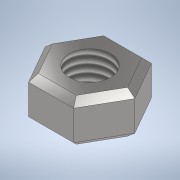
# Autodesk Inventor part: 6-luomu
Saved by Autodesk Inventor 2022 (Build 260153000, 153)
## iProperties
Created: 2023-01-24
Part Number: 6-luomu
Material: 不锈钢
Document SubType Name: Modeling
Designer: Lzy18
Density: 8 g/cm^3
Appearance: 半抛光
Author: Lzy18
Autodesk Inventor part; units mm, degrees
ref_plane "YZ Plane" through (0, 0, 0) normal (1, 0, 0) x (0, 1, 0)
ref_plane "XZ Plane" through (0, 0, 0) normal (0, 1, 0) x (-1, 0, 0)
ref_plane "XY Plane" through (0, 0, 0) normal (0, 0, 1) x (1, 0, 0)
sketch "草图1" plane through (0, 0, 0) normal (0, 1, 0) x (-1, 0, 0)
  line L0 (0, 0) -> (7.2, 0)
  line L1 (7.2, 0) -> (3.6254, -6.25)
  line L2 (3.6254, -6.25) -> (0, -6.25)
  line L3 (7.2, 0) -> (3.6254, 6.25)
  line L4 (3.6254, 6.25) -> (0, 6.25)
  line L5 (0, 0) -> (0, -6.25)
  line L6 (-7.2, 0) -> (-3.6254, -6.25)
  line L7 (-3.6254, -6.25) -> (0, -6.25)
  line L8 (-7.2, 0) -> (-3.6254, 6.25)
  line L9 (-3.6254, 6.25) -> (0, 6.25)
  dimension "d2" = 14.4
  dimension "d3" = 12.5
  constraints: 20 end point, 5 symmetric about line, 2 coincident, 2 horizontal, 1 vertical
  measures "d2" distance of L8.start L0.end
  measures "d3" distance of L4.end L2.end
extrude "拉伸1" add sketch "草图1" along normal blind 6.8
sketch "草图2" plane through (0, 6.8, 0) normal (0, 1, 0) x (1, 0, 0)
  circle A0 centre (0, 0) radius 6.25
  dimension "d6" = 12.5
  constraints: 1 centre point, 1 coincident
  measures "d6" diameter of A0
hole "孔1" at (0, 6.8, 0) direction (0, -1, 0) diameter 6.647 end through all thread size "M8x1.25" designation "M8" class "6H" standard "GB Metric profile"
chamfer "倒角3" distance 1 angle 45 12 edges at (0, 6.8, 6.25) (5.4127, 6.8, 3.125) (5.4127, 6.8, -3.125) (0, 6.8, -6.25) (-5.4127, 6.8, -3.125) (-5.4127, 6.8, 3.125) (5.4127, 0, 3.125) (5.4127, 0, -3.125) (0, 0, -6.25) (-5.4127, 0, -3.125) (-5.4127, 0, 3.125) (0, 0, 6.25)
